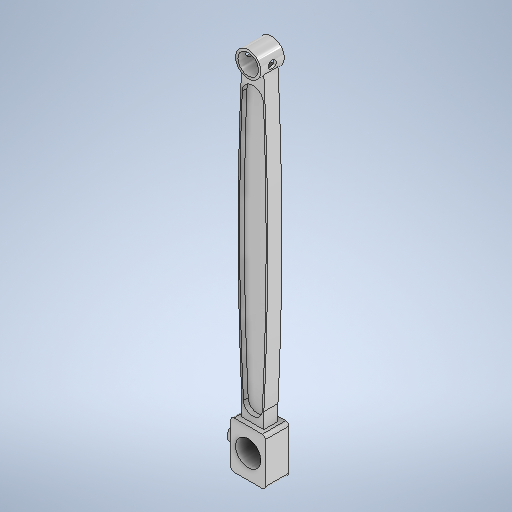
# Autodesk Inventor part: 2031
Saved by Autodesk Inventor 2025.1 (Build 291241000, 241)
## iProperties
Created: 2024-06-12
Part Number: 2031
Material: Aluminum 6061-AHC
Document SubType Name: Modeling
Designer: ffogue
Density: 2.7 g/cm^3
Appearance: Aluminium - dunkel
Author: ffogue
Autodesk Inventor part; units mm, degrees
note: some values were not read from the file. Chosen so that the rebuilt part matches the saved one: direction of "Bohrung2".
sketch "Skizze1" plane through (0, 0, 0) normal (0, 1, 0) x (-1, 0, 0)
  line L0 (0, 0) -> (22, 0)
  line L1 (22, 0) -> (22, -30)
  line L2 (22, -30) -> (0, -30)
  line L3 (0, -30) -> (0, 0)
  point P0 (0, -15)
  dimension "d0" = 30
  dimension "d1" = 22
  constraints: 8 end point, 2 parallel, 1 horizontal, 1 midpoint, 1 perpendicular
  measures "d0" distance between parallel lines of L2 L0
  measures "d1" distance from line of point (0, -15) L1
extrude "Extrusion1" add sketch "Skizze1" along normal blind 15
sketch "Skizze2" plane through (0, 15, 0) normal (0, 1, 0) x (1, 0, 0)
  circle A0 centre (-11, 15) radius 8
  line L0 (-22, 30) -> (-22, 0) projected
  line L1 (-22, 0) -> (0, 0) projected
  point P0 (-22, 15)
  point P1 (-11, 0)
  dimension "d4" = 16
  constraints: 2 midpoint, 1 centre point, 1 horizontal alignment, 1 vertical alignment
  measures "d4" diameter of A0
extrude "Extrusion2" cut sketch "Skizze2" against normal up to surface (15 mm away)
fillet "Rundung1" radius 2 4 edges at (-22, 7.5, -30) (0, 7.5, -30) (0, 7.5, 0) (-22, 7.5, 0)
sketch "Skizze3" plane through (-22, 0, -28) normal (-1, 0, 0) x (0, 0, 1)
  circle A0 centre (13, 7.5) radius 5
  line L0 (26, 15) -> (26, 0) projected
  line L1 (0, 0) -> (26, 0) projected
  point P0 (28, 0)
  point P1 (26, 7.5)
  point P2 (13, 0)
  dimension "d8" = 10
  constraints: 2 midpoint, 1 centre point, 1 horizontal alignment, 1 vertical alignment
  measures "d8" diameter of A0
extrude "Extrusion3" add sketch "Skizze3" along normal blind 5
sketch "Skizze4" plane through (-27, 7.5, -15) normal (-1, 0, 0) x (0, 0, 1)
  circle A0 centre (0, 0) radius 5 projected
  point P0 (15, -7.5)
  constraints: 1 coincident
hole "Bohrung1" at (-27, 7.5, -15) direction (1, 0, 0) diameter 4.917 depth 6 thread size "M6x1" class "6H" standard "ISO Metric profile"
ref_plane "Arbeitsebene1" through (0, 7.5, 0) normal (0, 1, 0) x (-1, 0, 0)
sketch "Skizze5" plane through (0, 7.5, 0) normal (0, 1, 0) x (-1, 0, 0)
  circle A0 centre (11, -15) radius 8 projected
  arc A1 (22, -2) -> (20, 0) centre (20, -2) ccw projected
  line L0 (22, -28) -> (22, -2) projected
  arc A2 (20, -30) -> (22, -28) centre (20, -28) ccw projected
  line L1 (2, -30) -> (20, -30) projected
  arc A3 (0, -28) -> (2, -30) centre (2, -28) ccw projected
  line L2 (0, -2) -> (0, -28) projected
  arc A4 (2, 0) -> (0, -2) centre (2, -2) ccw projected
  line L3 (20, 0) -> (2, 0) projected
  circle A5 centre (11, 200) radius 8
  point P0 (0, 0)
  dimension "d21" = 215
  dimension "d22" = 16
  constraints: 1 centre point, 1 vertical alignment
  measures "d21" distance of A0.centre A5.centre
  measures "d22" diameter of A5
extrude "Extrusion4" add sketch "Skizze5" along normal mid plane 15 contours A5
sketch "Skizze6" plane through (-11, 15, 200) normal (0, 1, 0) x (1, 0, 0)
  circle A0 centre (0, 0) radius 8 projected
  point P0 (11, 200)
  constraints: 1 coincident
hole "Bohrung2" at (-11, 15, 200) direction (0, -1, 0) diameter 13 depth 15
sketch "Skizze7" plane through (0, 7.5, 0) normal (0, 1, 0) x (-1, 0, 0)
  circle A0 centre (11, -15) radius 8 projected
  arc A1 (22, -2) -> (20, 0) centre (20, -2) ccw projected
  line L0 (22, -28) -> (22, -2) projected
  arc A2 (20, -30) -> (22, -28) centre (20, -28) ccw projected
  line L1 (2, -30) -> (20, -30) projected
  arc A3 (0, -28) -> (2, -30) centre (2, -28) ccw projected
  line L2 (0, -2) -> (0, -28) projected
  arc A4 (2, 0) -> (0, -2) centre (2, -2) ccw projected
  line L3 (20, 0) -> (2, 0) projected
  arc A5 (18, 10) -> (18, 196.127) centre (-1779.5926, 103.0635) ccw
  arc A6 (4, 196.127) -> (4, 10) centre (1801.5926, 103.0635) ccw
  line L4 (11, -30) -> (11, 0) construction
  line L5 (18, 0) -> (18, 10)
  line L6 (4, 0) -> (4, 10)
  line L7 (18, 196.127) -> (4, 196.127) construction
  circle A7 centre (11, 200) radius 8 projected
  arc A8 (4, 196.127) -> (18, 196.127) centre (11, 200) ccw
  point P0 (0, 0)
  point P1 (11, -15)
  point P2 (4, 5)
  point P3 (18, 5)
  dimension "d51" = 14
  dimension "d52" = 1800
  dimension "d53" = 1800
  dimension "d55" = 25
  dimension "d64" = 14
  constraints: 8 end point, 8 point on circle, 5 midpoint, 3 centre point, 2 point on line, 1 concentric, 1 horizontal, 1 horizontal alignment, 1 perpendicular, 1 symmetric about line, 1 vertical, 1 other
  measures "d51" distance of point (4, 5) point (18, 5)
  measures "d52" radius of A5
  measures "d53" radius of A6
  measures "d55" vertical distance of A0.centre L6.end
  measures "d64" distance of L7.start L7.end
extrude "Extrusion5" add sketch "Skizze7" along normal mid plane 9 contours L3 L6 A6 A7 A5 L5
sketch "Skizze8" plane through (0, 12, 0) normal (0, 1, 0) x (1, 0, 0)
  arc A0 (-17.7649, -180.33) -> (-4.2351, -180.33) centre (-11, -180.0392) ccw
  arc A1 (-18, -10) -> (-18, -196.127) centre (1779.5926, -103.0635) ccw projected
  arc A2 (-17, -9.6882) -> (-17.7649, -180.33) centre (1779.5926, -103.0635) ccw
  arc A3 (-4, -196.127) -> (-4, -10) centre (-1801.5926, -103.0635) ccw projected
  arc A4 (-4.2351, -180.33) -> (-5, -9.6882) centre (-1801.5926, -103.0635) ccw
  arc A5 (-5, -9.6882) -> (-17, -9.6882) centre (-11, -10) ccw
  circle A6 centre (-11, 15) radius 8 projected
  point P0 (0, 0)
  point P1 (-18, 0)
  point P2 (-18.2803, -197.1446)
  point P3 (-3.7197, -197.1446)
  point P4 (-4, 0)
  point P5 (-19.4068, -95)
  dimension "d38" = 25
  dimension "d40" = 12
  dimension "d41" = 85
  constraints: 9 point on circle, 4 centre point, 4 tangent, 1 vertical alignment
  measures "d38" distance of A6.centre A5.centre
  measures "d40" distance of A4.end A2.start
  measures "d41" vertical distance of point (-19.407, -95) A5.centre
extrude "Extrusion6" cut sketch "Skizze8" against normal blind 3 contours A2 A5 A4 A0
ref_plane "Arbeitsebene2" through (0, 7.5, 0) normal (0, 1, 0) x (-1, 0, 0)
mirror "Spiegeln1" about plane through (0, 7.5, 0) normal (0, 1, 0) of "Extrusion6"
ref_plane "Arbeitsebene3" through (-19, 0, 0) normal (1, 0, 0) x (0, 1, 0)
sketch "Skizze9" plane through (-19, 0, 0) normal (1, 0, 0) x (0, 1, 0)
  line L0 (0, 208) -> (15, 208) projected
  line L1 (0, 208) -> (0, 192) projected
  point P0 (0, 0)
  point P1 (7.5, 200)
  point P2 (7.5, 208)
  point P3 (0, 200)
  constraints: 2 midpoint, 1 horizontal alignment, 1 vertical alignment
hole "Bohrung3" at (-19, 7.5, 200) direction (1, 0, 0) diameter 4.917 end through all thread size "M6x1" class "6H" standard "ISO Metric profile"
equation "\"d53\" = d52"
